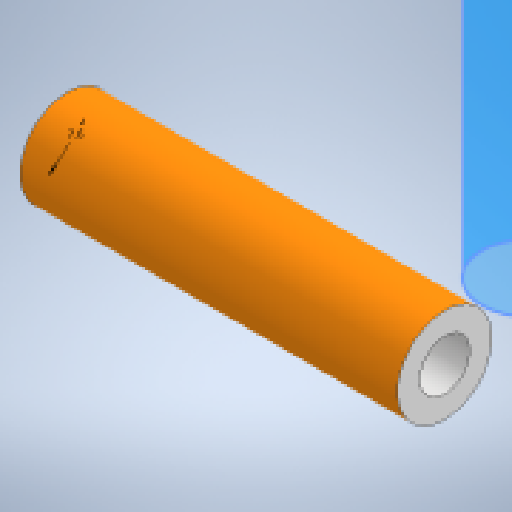
# Autodesk Inventor part: Stopper
Saved by Autodesk Inventor 2025.2 (Build 292293000, 293)
## iProperties
Created: 2025-03-13
Part Number: Stopper
Material: Generic
Document SubType Name: Modeling
Designer: baolo
Density: 1 g/cm^3
Appearance: Default
Author: baolo
Autodesk Inventor part; units mm, degrees
ref_plane "YZ Plane" through (0, 0, 0) normal (1, 0, 0) x (0, 1, 0)
ref_plane "XZ Plane" through (0, 0, 0) normal (0, 1, 0) x (-1, 0, 0)
ref_plane "XY Plane" through (0, 0, 0) normal (0, 0, 1) x (1, 0, 0)
sketch "Sketch1" plane through (0, 0, 0) normal (1, 0, 0) x (0, 1, 0)
  circle A0 centre (0, 0) radius 7.5
  dimension "d0" = 15
  constraints: 1 centre point, 1 coincident
  measures "d0" diameter of A0
extrude "Extrusion1" add sketch "Sketch1" along normal blind 60
sketch "Sketch2" plane through (0, 0, 0) normal (-1, 0, 0) x (0, 0, 1)
  point P0 (0, 0)
hole "Hole1" at (0, 0, 0) direction (1, 0, 0) diameter 8 end through all
sketch "Sketch3" plane through (0, 0, 0) normal (0, 1, 0) x (-1, 0, 0)
  line L0 (-60, -4) -> (0, -4) construction
  line L1 (0, -4) -> (-0.625, -2.9175) construction
  line L2 (-0.625, -2.9175) -> (-1.25, -4) construction
  line L3 (-1.25, -4) -> (-1.875, -5.0825) construction
  line L4 (-0.625, -2.9175) -> (-0.625, -4) construction
  line L5 (0, -4) -> (-0.5469, -3.0528)
  line L6 (-0.5469, -3.0528) -> (-0.7031, -3.0528)
  line L7 (-0.7031, -3.0528) -> (-1.25, -4)
  line L8 (-1.25, -4) -> (0, -4)
  point P0 (0, 0)
  dimension "d19" = 30
  dimension "d20" = 60
  dimension "d22" = 0.1562
  dimension "d31" = 1.25
  constraints: 16 end point, 5 point on line, 4 collinear, 2 perpendicular
  measures "d19" angle of L2 L4
  measures "d20" angle of L2 L1
  measures "d22" distance of L5.end L6.end
  measures "d31" distance of L2.end point (0, -4)
coil "Coil1" sketch "Sketch3" operation add axis through (-10, 0, 0) along (1, 0, 0) pitch 1.25 turns 40 hand right
sketch "Sketch4" plane through (0, 0, 0) normal (-1, 0, 0) x (0, 0, 1)
  circle A0 centre (0, 0) radius 3.8
  dimension "d32" = 7.6
  constraints: 1 centre point, 1 coincident
  measures "d32" diameter of A0
equation "\"d22\" = 0.125 * threadPitch"
equation "\"d31\" = threadPitch"
equation "\"d23\" = threadPitch"
equation "\"threadPitch\" = 1.25"
body "Solid1"
